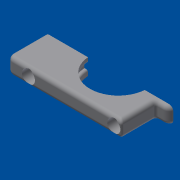
# Autodesk Inventor part: Prensa 30-12-2015
Saved by Autodesk Inventor 2015 (Build 190159000, 159)
## iProperties
Created: 2015-08-14
Part Number: Prensa 30-12-2015
Material: Genérico
Document SubType Name: Modeling
Designer: kelliton
Density: 1 g/cm^3
Appearance: Padrão
Author: kelliton
Autodesk Inventor part; units mm, degrees
ref_plane "YZ Plane" through (0, 0, 0) normal (1, 0, 0) x (0, 1, 0)
ref_plane "XZ Plane" through (0, 0, 0) normal (0, 1, 0) x (-1, 0, 0)
ref_plane "XY Plane" through (0, 0, 0) normal (0, 0, 1) x (1, 0, 0)
sketch "Prensa" plane through (0, 0, 0) normal (0, 0, 1) x (1, 0, 0)
  arc A0 (25.0501, 17) -> (44.9499, 17) centre (35, 18) ccw
  line L0 (0, 17) -> (25.0501, 17)
  line L1 (44.9499, 17) -> (63, 17)
  line L2 (0, 17) -> (0, -2)
  line L3 (0, -2) -> (63, -2)
  line L4 (63, -2) -> (63, 17)
  line L5 (63, -2) -> (56.5, -2)
  line L6 (56.5, -2) -> (56.5, 15)
  line L7 (56.5, 15) -> (63, 15)
  line L8 (63, 15) -> (63, -2)
  point P0 (-5.3446, 0)
  dimension "d13" = 63
  dimension "d27" = 19
  dimension "d28" = 63
  dimension "d40" = 6.5
  dimension "d41" = 17
  dimension "d47" = 35
  dimension "d48" = 20
  constraints: 18 end point, 3 perpendicular, 2 horizontal, 2 parallel, 2 point on circle, 1 centre point, 1 collinear, 1 vertical
  measures "d13" distance of L0.start L1.end
  measures "d27" distance of L0.start L2.end
  measures "d28" distance of L2.end L3.end
  measures "d40" distance of L6.end L7.end
  measures "d41" distance of L5.end L6.end
  measures "d47" distance from line of L2 A0.centre
  measures "d48" distance from line of L3 A0.centre
extrude "Extrusão1" add sketch "Prensa" along normal blind 8 contours A0 L1 L4 L7 L6 L3 L2 L0
sketch "Furo Passante" plane through (44.9499, 17, 0) normal (0, 1, 0) x (1, 0, 0)
  circle A0 centre (-34.2499, -4) radius 1.7
  circle A1 centre (7.7501, -4) radius 1.7
  line L0 (-44.9499, 0) -> (-44.9499, -8) projected
  line L1 (18.0501, -8) -> (0, -8) projected
  line L2 (-19.8997, -8) -> (-44.9499, -8) projected
  line L3 (18.0501, 0) -> (18.0501, -8) projected
  dimension "d16" = 3.4
  dimension "d17" = 3.4
  dimension "d18" = 10.7
  dimension "d19" = 42
  dimension "d20" = 4
  dimension "d21" = 4
  dimension "d60" = 10.3
  constraints: 2 centre point
  measures "d16" diameter of A0
  measures "d17" diameter of A1
  measures "d18" distance from line of A0.centre L0
  measures "d19" distance of A1.centre A0.centre
  measures "d20" distance from line of L1 A1.centre
  measures "d21" distance from line of L2 A0.centre
  measures "d60" distance from line of L3 A1.centre
extrude "Extrusão2" cut sketch "Furo Passante" against normal blind 20
sketch "Rebaixo Furo" plane through (0, -2, 0) normal (0, -1, 0) x (1, 0, 0)
  circle A0 centre (10.7, 4) radius 3.2
  circle A1 centre (52.7, 4) radius 3.2
  line L0 (56.5, 0) -> (0, 0) projected
  line L1 (0, 0) -> (0, 8) projected
  point P0 (63, 0)
  dimension "d31" = 6.4
  dimension "d32" = 6.4
  dimension "d33" = 4
  dimension "d34" = 4
  dimension "d35" = 10.7
  dimension "d36" = 42
  constraints: 2 centre point
  measures "d31" diameter of A0
  measures "d32" diameter of A1
  measures "d33" distance from line of L0 A0.centre
  measures "d34" distance from line of L0 A1.centre
  measures "d35" distance from line of L1 A0.centre
  measures "d36" distance of A0.centre A1.centre
extrude "Extrusão3" cut sketch "Rebaixo Furo" against normal blind 8
fillet "Arredondamento2" radius 3 1 edges at (63, 15, 4)
fillet "Arredondamento3" radius 1 1 edges at (56.5, 15, 4)
fillet "Arredondamento4" radius 1 1 edges at (56.5, -2, 4)
fillet "Arredondamento5" radius 3 1 edges at (0, -2, 4)
sketch "Esboço5" plane through (0, 0, 8) normal (0, 0, 1) x (1, 0, 0)
  circle A0 centre (35, 18) radius 14
  line L0 (3, -2) -> (55.5, -2) projected
  line L1 (0, 17) -> (0, 1) projected
  point P0 (0, 0)
  dimension "d49" = 28
  dimension "d50" = 20
  dimension "d51" = 35
  constraints: 1 centre point
  measures "d49" diameter of A0
  measures "d50" distance from line of L0 A0.centre
  measures "d51" distance from line of A0.centre L1
extrude "Extrusão4" cut sketch "Esboço5" against normal blind 8
ref_plane "Plano de trabalho1" through (0, 0, 4) normal (0, 0, 1) x (1, 0, 0)
sketch "Esboço6" plane through (0, 0, 4) normal (0, 0, 1) x (1, 0, 0)
  circle A0 centre (35, 18) radius 15.75
  line L0 (3, -2) -> (55.5, -2) projected
  line L1 (0, 17) -> (0, 1) projected
  point P0 (0, 0)
  dimension "d55" = 31.5
  dimension "d56" = 20
  dimension "d57" = 35
  constraints: 1 centre point
  measures "d55" diameter of A0
  measures "d56" distance from line of L0 A0.centre
  measures "d57" distance from line of A0.centre L1
extrude "Extrusão5" cut sketch "Esboço6" along normal mid plane 3
fillet "Arredondamento6" radius 2 2 edges at (51, 17, 4) (9, 17, 4)
fillet "Arredondamento7" radius 1 2 edges at (51, 6, 4) (9, 6, 4)
fillet "Arredondamento8" radius 2 16 edges at (29.25, -2, 8) (56.2071, -1.7071, 8) (56.5, 6.5, 8) (56.7929, 14.7071, 8) (58.8358, 15, 8) (61.9036, 15.5505, 8) (0.8787, -1.1213, 8) (0, 9, 8) (0.8787, -1.1213, 0) (0, 9, 0) (56.2071, -1.7071, 0) (56.5, 6.5, 0) (56.7929, 14.7071, 0) (58.8358, 15, 0) (61.9036, 15.5505, 0) (29.25, -2, 0)
fillet "Arredondamento9" radius 1 2 edges at (35, 4, 5.5) (35, 4, 2.5)
